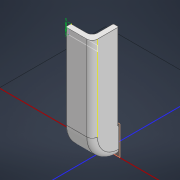
# Autodesk Inventor part: frame-foot
Saved by Autodesk Inventor 2021 (Build 250183000, 183)
## iProperties
Created: 2020-05-09
Part Number: frame-foot
Material: Generic
Document SubType Name: Modeling
Designer: Jonathan
Density: 1 g/cm^3
Appearance: Default
Author: Jonathan
Autodesk Inventor part; units mm, degrees
ref_plane "YZ Plane" through (0, 0, 0) normal (1, 0, 0) x (0, 1, 0)
ref_plane "XZ Plane" through (0, 0, 0) normal (0, 1, 0) x (-1, 0, 0)
ref_plane "XY Plane" through (0, 0, 0) normal (0, 0, 1) x (1, 0, 0)
ref_plane "Work Plane1" through (0, 0, 0) normal (0, 0, 1) x (1, 0, 0)
sketch "Sketch1" plane through (0, 0, 0) normal (0, 0, 1) x (1, 0, 0)
  arc A0 (12.5, 11.5) -> (11.5, 12.5) centre (11.5, 11.5) ccw projected
  line L0 (8.5, 12.5) -> (11.5, 12.5) projected
  arc A1 (8.5, 12.5) -> (7.5, 11.5) centre (8.5, 11.5) ccw projected
  line L1 (7.5, -2.5) -> (7.5, 11.5) projected
  arc A2 (2.5, -7.5) -> (7.5, -2.5) centre (2.5, -2.5) ccw projected
  line L2 (-11.5, -7.5) -> (2.5, -7.5) projected
  arc A3 (-11.5, -7.5) -> (-12.5, -8.5) centre (-11.5, -8.5) ccw projected
  line L3 (-12.5, -11.5) -> (-12.5, -8.5) projected
  arc A4 (-12.5, -11.5) -> (-11.5, -12.5) centre (-11.5, -11.5) ccw projected
  line L4 (7.5, -12.5) -> (-11.5, -12.5) projected
  arc A5 (7.5, -12.5) -> (12.5, -7.5) centre (7.5, -7.5) ccw projected
  line L5 (12.5, 11.5) -> (12.5, -7.5) projected
  point P0 (0, 0)
revolve "Revolution1" add sketch "Sketch1" angle 90 about axis through (8.5, 12.5, 0) along (-1, 0, 0)
sketch "Sketch2" plane through (8.5, 12.5, 0) normal (0, 1, 0) x (1, 0, 0)
  line L0 (4, -20) -> (4, -1) projected
  arc A0 (4, -1) -> (3, 0) centre (3, -1) ccw projected
  line L1 (3, 0) -> (0, 0) projected
  arc A1 (0, 0) -> (-1, -1) centre (0, -1) ccw projected
  line L2 (-1, -1) -> (-1, -15) projected
  arc A2 (-6, -20) -> (-1, -15) centre (-6, -15) ccw projected
  line L3 (-6, -20) -> (-20, -20) projected
  arc A3 (-20, -20) -> (-21, -21) centre (-20, -21) ccw projected
  line L4 (-21, -21) -> (-21, -24) projected
  arc A4 (-21, -24) -> (-20, -25) centre (-20, -24) ccw projected
  line L5 (-20, -25) -> (-1, -25) projected
  arc A5 (-1, -25) -> (4, -20) centre (-1, -20) ccw projected
  point P0 (-8.5, 0)
extrude "Extrusion1" add sketch "Sketch2" along normal up to surface (79.8139 mm away)
sketch "Sketch5" plane through (7.5, -12.5, 0) normal (0, 0, -1) x (-1, 0, 0)
  line L0 (20, 99.8139) -> (-1, 99.8139)
  line L1 (-1, 99.8139) -> (-1, 94.8139)
  line L2 (-1, 94.8139) -> (20, 94.8139)
  line L3 (20, 94.8139) -> (20, 99.8139)
  line L4 (20, 25) -> (20, 104.8139) projected
  line L5 (19, 104.8139) -> (5, 104.8139) projected
  point P0 (7.5, 12.5)
  point P1 (-1, 104.8139)
  dimension "d10" = 5
  dimension "d11" = 5
  constraints: 8 end point, 2 parallel, 2 point on line, 1 horizontal, 1 perpendicular
  measures "d10" distance between parallel lines of L5 L0
  measures "d11" distance between parallel lines of L0 L2
extrude "Extrusion4" add sketch "Sketch5" against normal up to next
sketch "Sketch6" plane through (-12.5, 82.3139, 0) normal (0, -1, 0) x (1, 0, 0)
  circle A0 centre (13.6397, 8.3297) radius 1.65
  circle A1 centre (6.1397, 8.3297) radius 1.65
  line L0 (13.6397, 8.3297) -> (6.1397, 8.3297) construction
  point P0 (12.5, 0)
  dimension "d14" = 7.5
  dimension "d15" = 3.3
  constraints: 2 centre point, 2 end point, 1 equal radius, 1 horizontal, 1 horizontal alignment
  measures "d14" distance of L0.end L0.start
  measures "d15" diameter of A0
body "Solid1"
